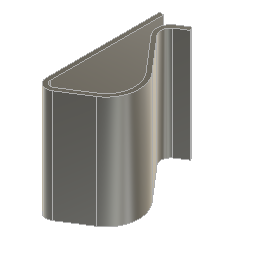
Glasses Clip v1 (Autodesk Fusion 360 design; units mm, degrees)
Autodesk Fusion 360 part; units mm, degrees
note: some values were not read from the file. Set by a fixed rule: which sketch regions a step uses.
sketch "Sketch1" plane through (0, 0, 0) normal (0, 0, 1) x (1, 0, 0)
  line L0 (0, 2.7263) -> (0, 35)
  line L1 (2.3029, 1.4592) -> (9.9175, 6.2842)
  arc A0 (9.9175, 6.2842) -> (11.71, 18.2478) centre (5.6356, 13.0418) ccw
  line L2 (11.71, 18.2478) -> (3.2204, 28.1536)
  arc A1 (3.9309, 34.0102) -> (3.2204, 28.1536) centre (6.2576, 30.7565) ccw
  line L3 (3.9309, 34.0102) -> (7.0243, 35.9704)
  line L4 (-1.2, 35) -> (0, 35)
  line L5 (7.0243, 35.9704) -> (7.6666, 34.9567)
  arc A2 (0, 2.7263) -> (2.3029, 1.4592) centre (1.5, 2.7263) ccw
  line L6 (4.6041, 33.0162) -> (7.6666, 34.9567)
  arc A3 (4.6041, 33.0162) -> (4.1316, 28.9345) centre (6.2576, 30.7565) ccw
  line L7 (12.6211, 19.0286) -> (4.1316, 28.9345)
  arc A4 (10.5598, 5.2706) -> (12.6211, 19.0286) centre (5.6356, 13.0418) ccw
  line L8 (2.9452, 0.4456) -> (10.5598, 5.2706)
  arc A5 (-1.2, 2.7263) -> (2.9452, 0.4456) centre (1.5, 2.7263) ccw
  line L9 (-1.2, 2.7263) -> (-1.2, 35)
  dimension "d1" = 35
  dimension "d2" = 8
  dimension "d3" = 4
  dimension "d4" = -1.2
  dimension "d7" = 1.5
  constraint vertical L0
  constraint tangent L1 A0
  constraint tangent A0 L2
  constraint tangent L2 A1
  constraint parallel L1 L3
  constraint perpendicular L0 L4
  constraint coincident origin L0
  constraint tangent L0 A2
  constraint tangent L1 A2
  measures "d1" distance of origin L0.end
  measures "d2" radius of A0
  measures "d3" radius of A1
  measures "d7" radius of A2
extrude "Extrude1" add sketch "Sketch1" along normal blind 32
named bodies: "glasses-clip"
